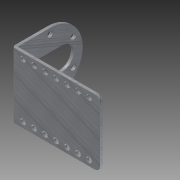
# Autodesk Inventor part: beslag
Saved by Autodesk Inventor 2012 (Build 160160000, 160)
## iProperties
Created: 2012-02-28
Part Number: beslag
Material: Default
Document SubType Name: Modeling
Designer: Grailas
Density: 1 g/cm^3
Author: Grailas
Autodesk Inventor part; units mm, degrees
ref_plane "YZ Plane" through (0, 0, 0) normal (1, 0, 0) x (0, 1, 0)
ref_plane "XZ Plane" through (0, 0, 0) normal (0, 1, 0) x (-1, 0, 0)
ref_plane "XY Plane" through (0, 0, 0) normal (0, 0, 1) x (1, 0, 0)
sketch "Sketch1" plane through (0, 0, 0) normal (0, 0, 1) x (1, 0, 0)
  line L0 (24.605, -18.795) -> (-24.605, -18.795)
  line L1 (-24.605, -18.795) -> (-24.605, 18.795)
  line L2 (-24.605, 18.795) -> (24.605, 18.795)
  line L3 (24.605, 18.795) -> (24.605, -18.795)
  line L4 (26.195, 20.385) -> (-26.195, 20.385)
  line L5 (-26.195, 20.385) -> (-26.195, 18.795)
  line L6 (-26.195, -20.385) -> (-24.605, -20.385)
  line L7 (26.195, -20.385) -> (26.195, 20.385)
  line L8 (24.605, -18.795) -> (24.605, -20.385)
  arc A0 (-26.195, -18.795) -> (-24.605, -20.385) centre (-24.605, -18.795) ccw
  line L9 (-24.605, -20.385) -> (24.605, -20.385)
  line L10 (-26.195, -18.795) -> (-26.195, -20.385)
  line L11 (-24.605, 18.795) -> (-26.195, 18.795)
  line L12 (-26.195, 18.795) -> (-26.195, -18.795)
  line L13 (24.605, -20.385) -> (26.195, -20.385)
  point P0 (0, 0)
  point P1 (0, -18.795)
  point P2 (-24.605, 0)
  dimension "d0" = 49.21
  dimension "d1" = 37.59
  dimension "d2" = 1.59
  constraints: 28 end point, 15 perpendicular, 8 parallel, 6 tangent, 2 horizontal alignment, 2 midpoint, 2 point on circle, 2 vertical alignment, 1 centre point, 1 horizontal, 1 point on line
  measures "d0" distance of L0.start L0.end
  measures "d1" distance of L0.end L1.end
  measures "d2" distance between parallel lines of L0 L6
extrude "Extrusion1" add sketch "Sketch1" against normal blind 37.59 contours L8 L9 A0 L12 L11 L1 L0
sketch "Sketch3" plane through (-24.605, -20.385, 0) normal (0, -1, 0) x (1, 0, 0)
  line L0 (0, -37.59) -> (49.21, -37.59) projected
  line L1 (49.21, 0) -> (49.21, -37.59) projected
  line L2 (0, 0) -> (49.21, 0) projected
  line L3 (0, 0) -> (0, -37.59) projected
  circle A0 centre (4.76, -3.175) radius 1.59
  circle A1 centre (11.11, -3.175) radius 1.59
  circle A2 centre (17.46, -3.175) radius 1.59
  circle A3 centre (23.81, -3.175) radius 1.59
  circle A4 centre (30.16, -3.175) radius 1.59
  circle A5 centre (36.51, -3.175) radius 1.59
  circle A6 centre (42.86, -3.175) radius 1.59
  arc A7 (49.21, -3.175) -> (46.035, 0) centre (46.035, -3.175) ccw
  line L4 (49.21, -18.795) -> (59.21, -18.795)
  circle A8 centre (4.76, -34.415) radius 1.59
  circle A9 centre (11.11, -34.415) radius 1.59
  circle A10 centre (17.46, -34.415) radius 1.59
  circle A11 centre (23.81, -34.415) radius 1.59
  circle A12 centre (30.16, -34.415) radius 1.59
  circle A13 centre (36.51, -34.415) radius 1.59
  circle A14 centre (42.86, -34.415) radius 1.59
  arc A15 (46.035, -37.59) -> (49.21, -34.415) centre (46.035, -34.415) ccw
  line L5 (46.035, -37.59) -> (49.21, -37.59)
  line L6 (49.21, -34.415) -> (49.21, -37.59)
  line L7 (49.21, -3.175) -> (49.21, 0)
  line L8 (46.035, 0) -> (49.21, 0)
  line L9 (-1.59, 0) -> (-1.59, -37.59) projected
  line L10 (-1.59, -37.59) -> (0, -37.59) projected
  line L11 (0, 0) -> (0, -37.59) projected
  line L12 (-1.59, 0) -> (0, 0) projected
  line L13 (-1.59, 0) -> (-1.59, -37.59) projected
  point P0 (24.605, 0)
  dimension "d12" = 6.35
  dimension "d13" = 6.35
  dimension "d14" = 6.35
  dimension "d15" = 6.35
  dimension "d16" = 6.35
  dimension "d17" = 6.35
  dimension "d18" = 6.35
  dimension "d19" = 3.18
  dimension "d20" = 15.62
  dimension "d21" = 10
  constraints: 16 centre point, 10 end point, 10 symmetric about line, 7 horizontal alignment, 6 equal radius, 6 tangent, 4 point on circle, 3 collinear, 2 perpendicular, 2 point on line, 1 midpoint, 8 other
  measures "d12" distance of A1.centre A0.centre
  measures "d13" distance of A2.centre A1.centre
  measures "d14" distance of A3.centre A2.centre
  measures "d15" distance of A4.centre A3.centre
  measures "d16" distance of A5.centre A4.centre
  measures "d17" distance of A6.centre A5.centre
  measures "d18" distance from line of L1 A6.centre
  measures "d19" diameter of A0
  measures "d20" vertical distance of A6.centre L4.start
  measures "d21" distance of L4.start L4.end
extrude "Extrusion2" cut sketch "Sketch3" against normal through all contours L3 L2 A7 L1 A15 L0 | L10 L9 L12 L3 keep common part
sketch "Sketch4" plane through (-26.195, -18.795, -37.59) normal (-1, 0, 0) x (0, 0, 1)
  line L0 (0, 37.59) -> (0, 0) projected
  line L1 (37.59, 0) -> (0, 0) projected
  line L2 (37.59, 37.59) -> (37.59, 0) projected
  line L3 (37.59, 37.59) -> (0, 37.59) projected
  line L4 (1.585, -1.59) -> (4.765, -1.59) projected
  line L5 (32.825, -1.59) -> (36.005, -1.59) projected
  line L6 (12.19, 11.785) -> (25.4, 11.785)
  line L7 (25.4, 11.785) -> (25.4, 25.805)
  line L8 (25.4, 25.805) -> (12.19, 25.805)
  line L9 (12.19, 25.805) -> (12.19, 11.785)
  arc A0 (25.4, 25.805) -> (12.19, 25.805) centre (18.795, 25.805) ccw
  arc A1 (12.19, 11.785) -> (25.4, 11.785) centre (18.795, 11.785) ccw
  arc A2 (18.795, 37.59) -> (0, 18.795) centre (18.795, 18.795) ccw
  line L10 (0, 18.795) -> (0, 37.59)
  line L11 (37.59, 37.59) -> (37.59, 18.795)
  line L12 (0, 37.59) -> (37.59, 37.59)
  circle A3 centre (18.795, 18.795) radius 15.5
  circle A4 centre (11.045, 32.2184) radius 1.625
  circle A5 centre (3.295, 18.795) radius 1.625
  circle A6 centre (11.045, 5.3716) radius 1.625
  circle A7 centre (26.545, 5.3716) radius 1.625
  circle A8 centre (34.295, 18.795) radius 1.625
  circle A9 centre (26.545, 32.2184) radius 1.625
  arc A10 (37.59, 18.795) -> (18.795, 37.59) centre (18.795, 18.795) ccw
  arc A11 (0, 18.795) -> (37.59, 18.795) centre (18.795, 18.795) ccw
  point P0 (3.295, 18.795)
  point P1 (26.545, 32.2184)
  point P2 (11.045, 5.3716)
  point P3 (34.295, 18.795)
  point P4 (26.545, 5.3716)
  dimension "d24" = 13.21
  dimension "d25" = 14.02
  dimension "d26" = 12.19
  dimension "d27" = 11.785
  dimension "d28" = 15.5
  dimension "d29" = 15.5
  dimension "d30" = 15.5
  dimension "d31" = 15.5
  dimension "d32" = 15.5
  dimension "d33" = 15.5
  dimension "d34" = 3.25
  dimension "d37" = 360
  constraints: 16 point on circle, 16 tangent, 14 end point, 12 centre point, 3 parallel, 2 coincident, 2 midpoint, 2 perpendicular, 1 collinear, 1 horizontal, 1 horizontal alignment, 13 other
  measures "d24" distance between parallel lines of L7 L9
  measures "d25" distance between parallel lines of L8 L6
  measures "d26" distance between parallel lines of L0 L9
  measures "d27" distance between parallel lines of L1 L6
  measures "d28" distance of point (26.545, 5.372) point (11.045, 5.372)
  measures "d29" distance of point (34.295, 18.795) point (26.545, 5.372)
  measures "d30" distance of A3.end point (34.295, 18.795)
  measures "d31" distance of point (11.045, 32.218) A3.end
  measures "d32" distance of point (11.045, 32.218) A3.start
  measures "d33" distance of point (11.045, 5.372) A3.start
  measures "d34" diameter of A4
extrude "Extrusion3" cut sketch "Sketch4" against normal through all contours L3 A2 L0 | L3 L2 A10 | L9 L8 L7 L6 | L6 A1 | A0 L8 | A3 A8 | A3 A8 | A9 A3 | A3 A9 | A7 A3 | A3 A7 | A4 A3 | A3 A4 | A6 A3 | A3 A6 | A5 A3 | A3 A5
equation "\"d13\" = d12"
equation "\"d14\" = d13"
equation "\"d15\" = d14"
equation "\"d16\" = d15"
equation "\"d17\" = d16"
equation "\"d18\" = d17"
equation "\"d29\" = d28"
equation "\"d30\" = d29"
equation "\"d31\" = d30"
equation "\"d32\" = d31"
equation "\"d33\" = d32"
body "Solid1"
